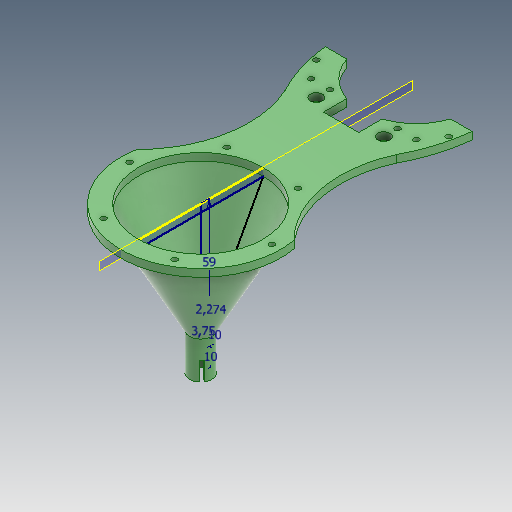
# Autodesk Inventor part: OneLensHolder
Saved by Autodesk Inventor 2020.3 (Build 243373000, 373)
## iProperties
Created: 2021-06-13
Part Number: OneLensHolder
Material: Generic
Document SubType Name: Modeling
Designer: Yusuf
Mass: 36.6691 g
Surface Area: 296.886 cm^2
Volume: 36.6691 cm^3
Density: 1 g/cm^3
Appearance: Smooth - Dark Forest Green
Author: Yusuf
Autodesk Inventor part; units mm, degrees
ref_plane "YZ Plane" through (0, 0, 0) normal (1, 0, 0) x (0, 1, 0)
ref_plane "XZ Plane" through (0, 0, 0) normal (0, 1, 0) x (-1, 0, 0)
ref_plane "XY Plane" through (0, 0, 0) normal (0, 0, 1) x (1, 0, 0)
sketch "Sketch1" plane through (0, 0, 0) normal (0, 1, 0) x (-1, 0, 0)
  line L0 (0, 0) -> (60, 0)
  line L1 (60, -81) -> (0, -81)
  line L2 (0, -81) -> (0, -40.5)
  line L3 (44.9096, -21.5055) -> (14.9096, -21.5055) construction
  line L4 (44.9096, -81) -> (44.9096, 0) construction
  line L5 (14.9096, 0) -> (14.9096, -81) construction
  circle A0 centre (39.9096, -73.5) radius 1.5
  circle A1 centre (39.9096, -7.5) radius 1.5
  circle A2 centre (19.9096, -7.5) radius 1.5
  circle A3 centre (19.9096, -73.5) radius 1.5
  line L6 (60, -40.5) -> (0, -40.5) construction
  line L7 (30, 0) -> (30, -81) construction
  circle A4 centre (30, -40.5) radius 24
  circle A5 centre (30, -40.5) radius 27.5
  circle A6 centre (57.1293, -36) radius 1.5
  circle A7 centre (57.1293, -45) radius 1.5
  circle A8 centre (25.5, -13.3707) radius 1.5
  circle A9 centre (34.5, -13.3707) radius 1.5
  circle A10 centre (2.8707, -45) radius 1.5
  circle A11 centre (2.8707, -36) radius 1.5
  circle A12 centre (34.5, -67.6293) radius 1.5
  circle A13 centre (25.5, -67.6293) radius 1.5
  arc A14 (60, -81) -> (60, 0) centre (-17.0125, -40.5) ccw
  arc A15 (-5.7831, -34.5157) -> (14.9096, -7.5073) centre (30, -40.5) ccw construction
  circle A16 centre (65.9998, -36) radius 1.5
  circle A17 centre (65.9998, -45) radius 1.5
  circle A18 centre (-5.9998, -45) radius 1.5
  circle A19 centre (-5.9998, -36) radius 1.5
  arc A20 (0, 0) -> (0, -81) centre (77.0125, -40.5) ccw
  line L8 (30, -40.5) -> (-3.3536, -73.8536) construction
  circle A21 centre (1.7157, -68.7843) radius 1.5
  circle A22 centre (11.8404, -76.1403) radius 1.5
  circle A23 centre (23.7426, -80.0075) radius 1.5
  circle A24 centre (36.2574, -80.0075) radius 1.5
  circle A25 centre (48.1596, -76.1403) radius 1.5
  circle A26 centre (58.2843, -68.7843) radius 1.5
  circle A27 centre (65.6403, -58.6596) radius 1.5
  circle A28 centre (69.5075, -46.7574) radius 1.5
  circle A29 centre (69.5075, -34.2426) radius 1.5
  circle A30 centre (65.6403, -22.3404) radius 1.5
  circle A31 centre (58.2843, -12.2157) radius 1.5
  circle A32 centre (48.1596, -4.8597) radius 1.5
  circle A33 centre (36.2574, -0.9925) radius 1.5
  circle A34 centre (23.7426, -0.9925) radius 1.5
  circle A35 centre (11.8404, -4.8597) radius 1.5
  circle A36 centre (1.7157, -12.2157) radius 1.5
  circle A37 centre (-5.6403, -22.3404) radius 1.5
  circle A38 centre (-9.5075, -34.2426) radius 1.5
  circle A39 centre (-9.5075, -46.7574) radius 1.5
  circle A40 centre (-5.6403, -58.6596) radius 1.5
  circle A41 centre (48.1596, -68.7843) radius 1.5
  circle A42 centre (48.1596, -12.2157) radius 1.5
  circle A43 centre (11.8404, -12.2157) radius 1.5
  circle A44 centre (11.8404, -68.7843) radius 1.5
  line L9 (56.4575, -33) -> (69.2906, -33)
  line L10 (37.5, -1.2094) -> (37.5, -14.0425)
  line L11 (37.5, -1.2094) -> (37.5, -14.0425)
  circle A45 centre (30, -40.5) radius 27.5
  line L12 (30, -81) -> (30, -0.5) construction
  line L13 (60, -33) -> (60, -81)
  arc A46 (60, -14.0425) -> (59.3249, -13.2961) centre (30, -40.5) ccw construction
  line L14 (55.807, -31) -> (69.4798, -31)
  circle A47 centre (48.1596, -4.8597) radius 3.25
  line L15 (51.4096, -4.8597) -> (51.4096, 0)
  line L16 (44.9096, -4.8597) -> (44.9096, 0)
  circle A48 centre (30, -40.5) radius 29.5
  line L17 (39.5, -12.5715) -> (39.5, 0)
  circle A49 centre (30, 75.5) radius 33.5
  line L18 (148.361, 0) -> (-88.361, 0) projected
  circle A50 centre (30, 75.5) radius 43
  arc A51 (37.7343, -1.2549) -> (13.1894, -4.2039) centre (30, -40.5) ccw
  arc A52 (-9.2451, -32.7657) -> (69.2451, -32.7657) centre (30, -40.5) ccw
  arc A53 (-9.2451, -32.7657) -> (69.2451, -32.7657) centre (30, -40.5) ccw construction
  arc A54 (37.7343, -1.2549) -> (13.1894, -4.2039) centre (30, -40.5) ccw construction
  line L19 (63.5, 75.5) -> (73, 75.5) construction
  circle A55 centre (68.25, 75.5) radius 1.5
  circle A56 centre (49.125, 108.6255) radius 1.5
  circle A57 centre (10.875, 108.6255) radius 1.5
  circle A58 centre (-8.25, 75.5) radius 1.5
  circle A59 centre (10.875, 42.3745) radius 1.5
  circle A60 centre (49.125, 42.3745) radius 1.5
  line L20 (4.193, -31) -> (-9.4798, -31)
  circle A61 centre (11.8404, -4.8597) radius 3.25
  line L21 (20.5, -12.5715) -> (20.5, 0)
  arc A62 (0, 0) -> (-12.2627, 67.5715) centre (-54.5436, 25) ccw
  arc A63 (72.2627, 67.5715) -> (60, 0) centre (114.5436, 25) ccw
  point P0 (29.9096, -21.5055)
  point P1 (30, -40.75)
  point P2 (-7.9036, 55.1945)
  point P3 (57.9285, -31)
  point P4 (2.0715, -31)
  point P5 (72.2627, 67.5715)
  point P6 (2.984, 42.0465)
  point P7 (57.016, 42.0465)
  dimension "d48" = 67
  dimension "d52" = 42
  dimension "d6" = 60
  dimension "d7" = 81
  dimension "d8" = 3
  dimension "d9" = 7.5
  dimension "d10" = 5
  dimension "d11" = 30
  dimension "d12" = 3
  dimension "d13" = 7.5
  dimension "d14" = 5
  dimension "d15" = 3
  dimension "d16" = 3
  dimension "d17" = 5
  dimension "d18" = 48
  dimension "d19" = 55
  dimension "d20" = 3
  dimension "d21" = 4.5
  dimension "d22" = 3
  dimension "d23" = 4.5
  dimension "d24" = 360
  dimension "d26" = 72.56
  dimension "d27" = 3
  dimension "d28" = 3
  dimension "d29" = 360
  dimension "d30" = 45
  dimension "d31" = 3
  dimension "d32" = 360
  dimension "d33" = 3
  dimension "d34" = 3
  dimension "d35" = 3
  dimension "d36" = 3
  dimension "d37" = 55
  dimension "d39" = 90
  dimension "d42" = 12.8331
  dimension "d43" = 12.8331
  dimension "d44" = 2
  dimension "d45" = 6.5
  dimension "d46" = 2
  dimension "d47" = 2
  dimension "d49" = 30
  dimension "d57" = 3
  dimension "d60" = 360
  dimension "d84" = 4.75
  dimension "d85" = 60
  dimension "d86" = 25
  constraints: 56 centre point, 42 end point, 38 point on circle, 12 point on line, 9 coincident, 9 horizontal alignment, 8 symmetric about line, 7 midpoint, 7 vertical alignment, 5 perpendicular, 3 horizontal, 3 parallel, 2 collinear, 2 tangent, 107 other
  measures "d6" distance of L1.start L2.start
  measures "d7" distance of L0.end L1.start
  measures "d8" diameter of A0
  measures "d9" distance from line of A0.centre L1
  measures "d10" distance from line of L4 A0.centre
  measures "d11" distance between parallel lines of L5 L4
  measures "d12" diameter of A1
  measures "d13" distance from line of L0 A1.centre
  measures "d14" distance from line of L4 A1.centre
  measures "d15" diameter of A2
  measures "d16" diameter of A3
  measures "d17" distance from line of L5 A2.centre
  measures "d18" diameter of A4
  measures "d19" diameter of A5
  measures "d20" diameter of A6
  measures "d21" distance from line of A6.centre L6
  measures "d22" diameter of A7
  measures "d23" distance from line of L6 A7.centre
  measures "d26" diameter of A15
  measures "d27" diameter of A16
  measures "d28" diameter of A17
  measures "d30" angle of L7 L8
  measures "d31" diameter of A21
  measures "d33" diameter of A41
  measures "d34" diameter of A42
  measures "d35" diameter of A43
  measures "d36" diameter of A44
  measures "d37" diameter of A45
  measures "d39" angle of L10 L9
  measures "d42" distance of L9.start L9.end
  measures "d43" distance of L10.start L10.end
  measures "d44" distance between parallel lines of L14 L9
  measures "d45" diameter of A47
  measures "d46" distance between parallel lines of L10 L17
  measures "d49" horizontal distance of L0.start A51.centre
  measures "d57" diameter of A55
  measures "d84" distance of L19.start A55.centre
  measures "d85" radius of A62
  measures "d86" vertical distance of L0.start A62.centre
extrude "Extrusion1" add sketch "Sketch1" along normal blind 4 contours A62 A50 A63 L0 A33 A34 | L0 L21 A2 A48 L20 A20 | A62 A50 A63 | A34 L0 | L21 A2 | A14 L14 A48 L17 A1 L0 L16 A47 L15 | A33 L0 | L15 A47 L16 L0 | L17 A1 picked at (20.0279, -7.9174) picked at (39.7286, -7.0086)
ref_plane "Work Plane1" through (-30, 0, -12.5715) normal (-1, 0, 0) x (0, 0, 1)
sketch "Sketch3" plane through (-30, 0, -12.5715) normal (-1, 0, 0) x (0, 0, 1)
  line L0 (54.5715, 0) -> (84.3215, -55)
  line L1 (54.5715, 0) -> (121.5715, 0) projected
  line L2 (121.5715, 0) -> (54.5715, 0)
  line L3 (54.5715, 4) -> (121.5715, 4) projected
  line L4 (88.0715, 4) -> (88.0715, -55)
  line L5 (84.3215, -55) -> (82.0477, -55)
  line L6 (82.0477, -55) -> (52.2977, 0)
  line L7 (52.2977, 0) -> (54.5715, 0)
  line L8 (84.3215, -55) -> (84.3215, -65)
  line L9 (82.0477, -55) -> (82.0477, -65)
  line L10 (84.3215, -65) -> (82.0477, -65)
  line L11 (84.3215, -65) -> (84.3215, -75)
  line L12 (84.3215, -75) -> (82.0477, -75)
  line L13 (82.0477, -75) -> (82.0477, -65)
  point P0 (12.5715, 0)
  point P1 (88.0715, 0)
  dimension "d88" = 59
  dimension "d89" = 3.75
  dimension "d94" = 10
  dimension "d96" = 2.2738
  dimension "d98" = 10
  constraints: 24 end point, 4 vertical, 3 parallel, 2 horizontal, 2 midpoint, 2 perpendicular
  measures "d88" distance of L4.start L4.end
  measures "d89" distance of L4.end L0.end
  measures "d94" distance of L5.end L9.end
  measures "d96" distance of L5.end L0.end
  measures "d98" distance of L8.end L11.end
revolve "Revolution4" add sketch "Sketch3" angle 360 about axis through (-30, 4, 75.5) along (0, -1, 0) contours L0 L5 L6 L7 | L8 L10 L9 L5
revolve "Revolution5" add sketch "Sketch3" angle 100 about axis through (-30, 4, 75.5) along (0, 1, 0) contours L11 L12 L13 L10
pattern_circular "Circular Pattern3" count 3 over 360 about axis through (-30, -60, 75.5) along (0, 1, 0) of "Revolution5"
equation "\"d11\" = 0.5 * d6"
equation "\"d12\" = d8"
equation "\"d15\" = d8"
equation "\"d16\" = d8"
equation "\"d22\" = d8"
equation "\"d27\" = d8"
equation "\"d28\" = d8"
equation "\"d31\" = d8"
equation "\"d33\" = d8"
equation "\"d34\" = d8"
equation "\"d35\" = d8"
equation "\"d36\" = d8"
body "Solid1"
